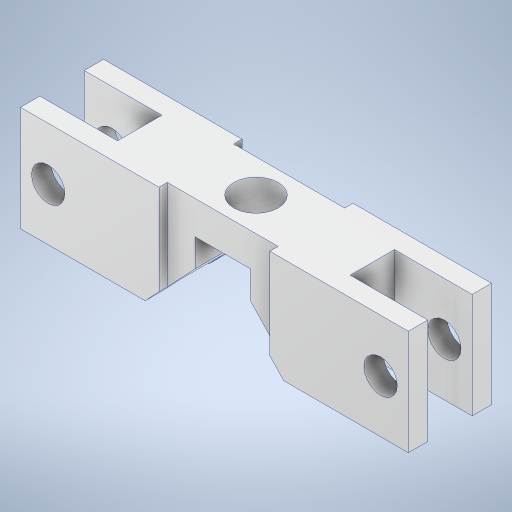
# Autodesk Inventor part: Belka
Saved by Autodesk Inventor 2024 (Build 280153000, 153)
## iProperties
Created: 2024-04-13
Part Number: Belka
Material: Aluminum 6061
Document SubType Name: Sheet Metal
Designer: HP
Density: 2.7 g/cm^3
Sheet Metal Rule: Default
Appearance: Aluminum - Flat
Author: HP
Autodesk Inventor part; units mm, degrees
ref_plane "YZ Plane" through (0, 0, 0) normal (1, 0, 0) x (0, 1, 0)
ref_plane "XZ Plane" through (0, 0, 0) normal (0, 1, 0) x (-1, 0, 0)
ref_plane "XY Plane" through (0, 0, 0) normal (0, 0, 1) x (1, 0, 0)
sketch "Sketch1" plane through (0, 0, 0) normal (0, 0, 1) x (1, 0, 0)
  line L0 (0, 0) -> (-5, 0)
  line L1 (0, 0) -> (5, 0)
  line L2 (-5, 0) -> (-5, -4) construction
  line L3 (-5, -4) -> (-23.8125, -4) construction
  line L4 (-5, 0) -> (10, 0) construction
  line L5 (0, -6.9282) -> (-35, -6.9282) construction
  line L6 (-12.5, -12.9904) -> (-35, -12.9904)
  line L7 (-23.8125, -4) -> (-23.8125, -8) construction
  line L8 (-35, -12.9904) -> (-35, -8)
  line L9 (-35, 0) -> (-35, 6)
  line L10 (-35, 6) -> (0, 6)
  line L11 (0, 6) -> (0, 0) construction
  line L12 (0, 0) -> (5, 0)
  line L13 (12.5, -12.9904) -> (35, -12.9904)
  line L14 (35, -12.9904) -> (35, -8)
  line L15 (35, 0) -> (35, 6)
  line L16 (35, 6) -> (0, 6)
  line L17 (-5, 0) -> (-5, -5)
  line L18 (-5, -5) -> (-12.5, -12.9904)
  line L19 (5, 0) -> (5, -5)
  line L20 (5, -5) -> (12.5, -12.9904)
  line L21 (-25, 0) -> (-21, 0)
  line L22 (-35, 0) -> (-35, -8)
  line L23 (35, 0) -> (35, -8)
  dimension "d0" = 5
  dimension "d1" = 5
  dimension "d2" = 4
  dimension "d3" = 15
  dimension "d5" = 35
  dimension "d10" = 6
  dimension "d24" = 5
  dimension "d25" = 5
  dimension "d27" = 4
  constraints: 48 end point, 8 vertical, 7 horizontal, 5 symmetric about line, 3 point on line, 1 perpendicular
  measures "d0" distance of L0.start L0.end
  measures "d1" distance of L0.start L1.end
  measures "d2" distance of L0.end L2.end
  measures "d3" distance of L0.end L6.start
  measures "d5" distance of L5.start L5.end
  measures "d10" distance of L9.start L9.end
  measures "d24" distance of L0.end L17.end
  measures "d25" distance of L1.end L19.end
  measures "d27" distance of L21.start L21.end
extrude "Extrusion1" add sketch "Sketch1" along normal mid plane 15
sketch "Sketch5" plane through (-35, 6, 7.5) normal (0, 1, 0) x (1, 0, 0)
  circle A0 centre (35, 7.5) radius 2 construction
  line L0 (35, 7.5) -> (35, 13.5) construction
  line L1 (35, 7.5) -> (25, 7.5) construction
  line L2 (35, 13.5) -> (25, 13.5)
  line L3 (25, 13.5) -> (25, 1.5)
  line L4 (25, 1.5) -> (45, 1.5)
  line L5 (45, 1.5) -> (45, 13.5)
  line L6 (45, 13.5) -> (35, 13.5)
  line L7 (25, 13.5) -> (25, 15)
  line L8 (0, 15) -> (70, 15) projected
  line L9 (45, 13.5) -> (45, 15)
  line L10 (45, 15) -> (25, 15)
  line L11 (25, 1.5) -> (25, 0)
  line L12 (25, 0) -> (45, 0)
  line L13 (40, 0) -> (47.5, 0) projected
  line L14 (45, 1.5) -> (45, 0)
  dimension "d40" = 6
  dimension "d41" = 10
  dimension "d42" = 12
  dimension "d43" = 20
  dimension "d44" = 12
  constraints: 26 end point, 6 point on line, 2 horizontal, 2 perpendicular, 2 vertical, 1 collinear, 1 parallel
  measures "d40" distance of L0.start L0.end
  measures "d41" distance of L0.start L1.end
  measures "d42" distance of L2.end L3.end
  measures "d43" distance of L3.end L4.end
  measures "d44" distance of L4.end L5.end
extrude "Extrusion5" cut sketch "Sketch5" against normal blind 18 contours L2 L7 L8 L9 L6 | L4 L14 L12 L11
sketch "Sketch6" plane through (35, 6, 7.5) normal (0, 1, 0) x (1, 0, 0)
  circle A0 centre (-35, 7.5) radius 4
  dimension "d47" = 8
  constraints: 1 centre point, 1 coincident
  measures "d47" diameter of A0
extrude "Extrusion6" cut sketch "Sketch6" against normal blind 6
sketch "Sketch7" plane through (35, 6, 7.5) normal (0, 1, 0) x (1, 0, 0)
  line L0 (-35, 7.5) -> (-65, 7.5) construction
  line L1 (-65, 7.5) -> (-65, 11.5) construction
  line L2 (-65, 11.5) -> (-65, 3.5) construction
  line L3 (-65, 3.5) -> (-70, 3.5)
  line L4 (-70, 15) -> (-70, 0) projected
  line L5 (-70, 3.5) -> (-70, 11.5)
  line L6 (-70, 11.5) -> (-65, 11.5)
  line L7 (-70, 11.5) -> (-65, 11.5)
  line L8 (-70, 11.5) -> (-56, 11.5)
  line L9 (-56, 11.5) -> (-56, 3.5)
  line L10 (-56, 3.5) -> (-70, 3.5)
  circle A0 centre (-35, 7.5) radius 4 construction
  line L11 (-35, 7.5) -> (-35, 1.5875) construction
  line L12 (0, 15) -> (0, 0)
  line L13 (0, 11.5) -> (-14, 11.5)
  line L14 (-14, 11.5) -> (-14, 3.5)
  line L15 (-14, 3.5) -> (0, 3.5)
  dimension "d50" = 30
  dimension "d51" = 4
  dimension "d52" = 8
  dimension "d53" = 14
  constraints: 30 end point, 6 symmetric about line, 4 point on line, 3 perpendicular, 3 vertical, 2 collinear, 1 horizontal
  measures "d50" distance of L0.start L0.end
  measures "d51" distance of L0.end L1.end
  measures "d52" distance of L1.end L2.end
  measures "d53" distance of L5.end L8.end
extrude "Extrusion7" cut sketch "Sketch7" against normal blind 19
sketch "Sketch8" plane through (0, 0, 7.5) normal (0, 0, 1) x (1, 0, 0)
  line L0 (0, 0) -> (-30, 0) construction
  line L1 (-21, 6) -> (-35, 6) construction
  line L2 (-30, 6) -> (-30, -3.5) construction
  line L3 (-30, 6) -> (-20.5, 6) construction
  circle A0 centre (-30, -3.5) radius 3
  line L4 (0, 0) -> (0, -2.1213) construction
  circle A1 centre (30, -3.5) radius 3
  dimension "d56" = 30
  dimension "d57" = 9.5
  dimension "d58" = 90
  dimension "d59" = 6
  constraints: 8 end point, 2 centre point, 2 horizontal, 2 perpendicular, 1 coincident, 1 point on line, 1 symmetric about line, 1 vertical, 1 other
  measures "d56" distance of L0.start L0.end
  measures "d57" distance of L2.start L2.end
  measures "d58" angle of L2 L3
  measures "d59" diameter of A0
extrude "Extrusion8" cut sketch "Sketch8" against normal blind 15
sketch "Sketch9" plane through (-35, -12.9904, -7.5) normal (0, -1, 0) x (1, 0, 0)
  line L0 (14, 3.5) -> (14, 11.5) construction
  line L1 (14, 11.5) -> (14, 11.5) construction
  line L2 (14, 11.5) -> (25.4, 11.5)
  line L3 (25.4, 11.5) -> (25.4, 3.5)
  line L4 (25.4, 3.5) -> (14, 3.5)
  line L5 (35, 7.5) -> (35, 13.3991) construction
  line L6 (14, 11.5) -> (14, 3.5)
  line L7 (56, 3.5) -> (56, 11.5) construction
  line L8 (56, 11.5) -> (44.6, 11.5)
  line L9 (44.6, 11.5) -> (44.6, 3.5)
  line L10 (44.6, 3.5) -> (56, 3.5)
  line L11 (56, 3.5) -> (56, 11.5)
  dimension "d62" = 0
  dimension "d63" = 90
  dimension "d64" = 8
  constraints: 22 end point, 6 symmetric about line, 4 point on line, 2 collinear, 2 perpendicular, 1 vertical
  measures "d62" distance of L0.end L1.end
  measures "d63" angle of L2 L1
  measures "d64" distance of L2.end L3.end
extrude "Extrusion9" cut sketch "Sketch9" against normal blind 3
equation "\"BendRadius\" = Thickness"
equation "\"BendReliefWidth\" = Thickness"
equation "\"BendReliefDepth\" = 0.5 * Thickness"
equation "\"CornerReliefSize\" = 4 * Thickness"
equation "\"MinimumRemnant\" = 2 * Thickness"
equation "\"TransitionRadius\" = BendRadius"
equation "\"JacobiRadiusSize\" = BendRadius"
equation "\"GapSize\" = Thickness"
equation "\"Thickness\" = 3.048"
body "Solid1"
